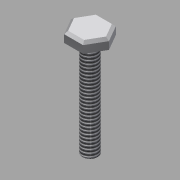
# Autodesk Inventor part: Bolt
Saved by Autodesk Inventor 2013 (Build 170138000, 138)
## iProperties
Created: 2013-01-18
Part Number: Bolt
Material: Aluminum 6061-AHC
Document SubType Name: Modeling
Designer: Naphat
Density: 1 g/cm^3
Author: Naphat
Autodesk Inventor part; units mm, degrees
ref_plane "YZ Plane" through (0, 0, 0) normal (1, 0, 0) x (0, 1, 0)
ref_plane "XZ Plane" through (0, 0, 0) normal (0, 1, 0) x (-1, 0, 0)
ref_plane "XY Plane" through (0, 0, 0) normal (0, 0, 1) x (1, 0, 0)
sketch "Sketch1" plane through (0, 0, 0) normal (0, 1, 0) x (-1, 0, 0)
  circle A0 centre (0, 0) radius 3
  dimension "d0" = 6
  constraints: 1 centre point, 1 coincident
  measures "d0" diameter of A0
extrude "Extrusion1" add sketch "Sketch1" along normal blind 39
sketch "Sketch2" plane through (0, 39, 0) normal (0, 1, 0) x (1, 0, 0)
  line L0 (-3.7501, -6.4954) -> (-7.5003, 0)
  line L1 (-7.5003, 0) -> (-3.7501, 6.4954)
  line L2 (-7.5003, 0) -> (0, 0) construction
  line L3 (-3.7501, 6.4954) -> (3.7501, 6.4954)
  line L4 (3.7501, 6.4954) -> (7.5003, 0)
  line L5 (3.7501, -6.4954) -> (7.5003, 0)
  line L6 (3.7501, -6.4954) -> (-3.7501, 6.4954) construction
  line L7 (3.7501, 6.4954) -> (-3.7501, -6.4954) construction
  line L8 (7.5003, 0) -> (-7.5003, 0) construction
  line L9 (3.7501, -6.4954) -> (-3.7501, -6.4954)
  dimension "d13" = 7.5003
  dimension "d18" = 7.5003
  dimension "d19" = 60
  dimension "d20" = 7.5003
  dimension "d21" = 120
  dimension "d22" = 120
  constraints: 20 end point, 4 parallel, 1 equal length, 1 horizontal
  measures "d13" distance of L0.start L0.end
  measures "d18" distance of L0.end L1.end
  measures "d19" angle of L2 L1
  measures "d20" distance of L3.end L4.end
  measures "d21" angle of L4 L3
  measures "d22" angle of L3 L1
extrude "Extrusion2" add sketch "Sketch2" along normal blind 4
thread "Thread2" size "1/4-20 UNC" class "2A" standard "ANSI Unified Screw Threads" full length
chamfer "Chamfer1" distance 1 angle 45 6 edges at (0, 43, 6.4954) (5.6252, 43, 3.2477) (5.6252, 43, -3.2477) (0, 43, -6.4954) (-5.6252, 43, -3.2477) (-5.6252, 43, 3.2477)
equation "\"d13\" = d9"
equation "\"d18\" = d13"
equation "\"d20\" = d9"
equation "\"d9\" = 7.500278"
body "Solid1"
